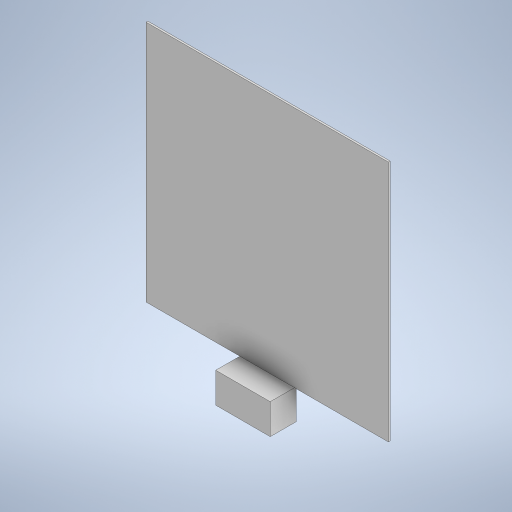
# Autodesk Inventor part: basicdifuserthin
Saved by Autodesk Inventor 2023 (Build 270158000, 158)
## iProperties
Created: 2022-05-18
Part Number: basicdifuserthin
Material: Generisch
Document SubType Name: Modeling
Designer: Tim Stechel
Density: 1 g/cm^3
Appearance: Vorgabe
Author: Tim Stechel
Autodesk Inventor part; units mm, degrees
ref_plane "YZ Plane" through (0, 0, 0) normal (1, 0, 0) x (0, 1, 0)
ref_plane "XZ Plane" through (0, 0, 0) normal (0, 1, 0) x (-1, 0, 0)
ref_plane "XY Plane" through (0, 0, 0) normal (0, 0, 1) x (1, 0, 0)
sketch "Skizze1" plane through (0, 0, 0) normal (0, 0, 1) x (1, 0, 0)
  line L0 (-20, 20) -> (20, 20)
  line L1 (20, 20) -> (20, -20)
  line L2 (20, -20) -> (-20, -20)
  line L3 (-20, -20) -> (-20, 20)
  line L4 (0, 20) -> (0, -20)
  line L5 (-20, 0) -> (20, 0)
  point P0 (0, 0)
  point P1 (0, 0)
  point P2 (-20, 0)
  point P3 (0, 0)
  point P4 (20, 0)
  dimension "d1" = 40
  dimension "d2" = 40
  constraints: 12 end point, 6 midpoint, 2 coincident, 2 parallel, 2 perpendicular, 1 horizontal, 2 other
  measures "d1" distance of L0.start L0.end
  measures "d2" distance of L0.end L1.end
extrude "Extrusion1" add sketch "Skizze1" along normal blind 0.3
sketch "Skizze2" plane through (0, 0, 0.3) normal (0, 0, 1) x (1, 0, 0)
  line L0 (-20, -20) -> (20, -20) projected
  line L1 (-4.5, -20) -> (4.5, -20)
  line L2 (4.5, -20) -> (4.5, -25)
  line L3 (4.5, -25) -> (-4.5, -25)
  line L4 (-4.5, -25) -> (-4.5, -20)
  line L5 (0, -20) -> (0, -25)
  point P0 (0, 0)
  dimension "d5" = 5
  dimension "d6" = 9
  constraints: 10 end point, 2 midpoint, 2 parallel, 2 perpendicular, 1 horizontal, 1 point on line, 1 other
  measures "d5" distance of L1.end L2.end
  measures "d6" distance of L2.end L3.end
extrude "Extrusion2" add sketch "Skizze2" along normal blind 4 and the other way blind 0.3
equation "\"d2\" = d1"
